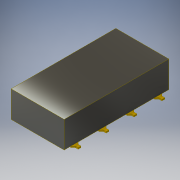
# Autodesk Inventor part: MC_YY101
Saved by Autodesk Inventor 2016 (Build 200138000, 138)
## iProperties
Created: 2016-08-30
Part Number: MC_YY101
Material: Generic
Document SubType Name: Modeling
Designer: jfixelle
Density: 1 g/cm^3
Appearance: Silver
Author: jfixelle
Autodesk Inventor part; units mm, degrees
ref_plane "YZ Plane" through (0, 0, 0) normal (1, 0, 0) x (0, 1, 0)
ref_plane "XZ Plane" through (0, 0, 0) normal (0, 1, 0) x (-1, 0, 0)
ref_plane "XY Plane" through (0, 0, 0) normal (0, 0, 1) x (1, 0, 0)
sketch "Sketch1" plane through (0, 0, 0) normal (0, 1, 0) x (-1, 0, 0)
  line L0 (4.825, 9.525) -> (-4.825, 9.525)
  line L1 (-4.825, 9.525) -> (-4.825, -9.525)
  line L2 (-4.825, -9.525) -> (4.825, -9.525)
  line L3 (4.825, -9.525) -> (4.825, 9.525)
  point P0 (0, 0)
  dimension "d0" = 9.65
  dimension "d1" = 4.825
  dimension "d2" = 19.05
  dimension "d3" = 9.525
  constraints: 8 end point, 2 parallel, 1 horizontal, 1 perpendicular
  measures "d0" distance of L0.start L0.end
  measures "d1" distance from line of point (0, 0) L3
  measures "d2" distance of L2.end L0.start
  measures "d3" distance from line of point (0, 0) L2
extrude "Extrusion1" add sketch "Sketch1" along normal blind 4.83
sketch "Sketch2" plane through (0, 0, 0) normal (0, -1, 0) x (1, 0, 0)
  line L0 (5.715, 8.25) -> (3.935, 8.25)
  line L1 (3.935, 8.25) -> (3.935, 6.98)
  line L2 (3.935, 6.98) -> (5.715, 6.98)
  line L3 (5.715, 6.98) -> (5.715, 8.25)
  line L4 (-4.825, 9.525) -> (4.825, 9.525) projected
  line L5 (4.825, 9.525) -> (4.825, -9.525) projected
  line L6 (5.715, 7.87) -> (5.205, 7.87)
  line L7 (5.205, 7.36) -> (5.715, 7.36)
  line L8 (5.715, 7.36) -> (5.715, 7.87)
  line L9 (4.825, 8.25) -> (5.205, 7.87)
  line L10 (5.205, 7.36) -> (4.825, 6.98)
  point P0 (0, 0)
  dimension "d6" = 1.27
  dimension "d7" = 1.78
  dimension "d8" = 5.715
  dimension "d9" = 1.275
  dimension "d10" = 0.51
  dimension "d11" = 0.38
  dimension "d12" = 45
  dimension "d13" = 45
  constraints: 18 end point, 3 parallel, 3 point on line, 2 horizontal, 2 midpoint, 1 perpendicular
  measures "d6" distance of L2.end L0.start
  measures "d7" distance of L1.end L2.end
  measures "d8" distance from line of point (0, 0) L3
  measures "d9" distance between parallel lines of L0 L4
  measures "d10" distance between parallel lines of L7 L6
  measures "d11" distance between parallel lines of L0 L6
  measures "d12" angle of L2 L10
  measures "d13" angle of L0 L9
extrude "Extrusion2" add sketch "Sketch2" along normal blind 0.25 contours L5 L2 L1 L0 | L9 L6 L3 L7 L10 L5
pattern_linear "Rectangular Pattern1" count 4 spacing 5.08 along (0, 0, -1) of "Extrusion2"
mirror "Mirror1" about plane through (0, 0, 0) normal (1, 0, 0) of "Extrusion2", "Rectangular Pattern1"
body "Solid1"
